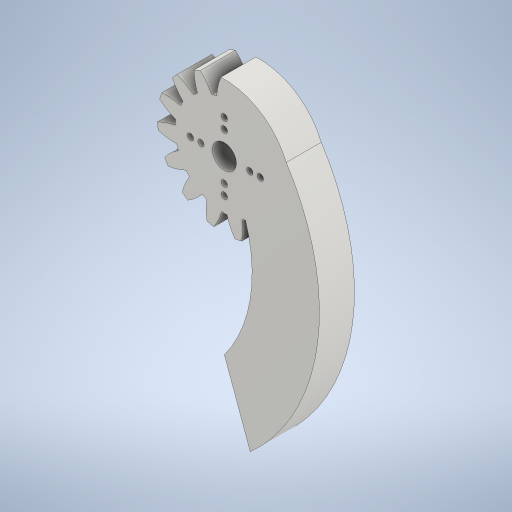
# Autodesk Inventor part: Spur Gear22
Saved by Autodesk Inventor 2024 (Build 280153000, 153)
## iProperties
CustomPartVersion: 0
Created: 2023-09-24
Part Number: Spur Gear22
Material: Steel
Document SubType Name: Modeling
Designer: jebes windows
Categories: <?xml version="1.0" encoding="UTF-16"?> <MemberInstance><Categories><FamilyTemplate><FamilyTemplateParameter ValueType="xs:double" Id="1" ObjectReferenceKey="da_z" ObjectType="kUserParameterObject"/><FamilyTemplateParameter ValueType="xs:double" Id="2" ObjectReferenceKey="da_b" ObjectType="kUserParameterObject"/><FamilyTemplateParameter ValueType="xs:double" Id="3" ObjectReferenceKey="da_beta" ObjectType="kUserParameterObject"/><FamilyTemplateParameter ValueType="xs:double" Id="4" ObjectReferenceKey="da_da" ObjectType="kUserParameterObject"/><FamilyTemplateParameter ValueType="xs:double" Id="5" ObjectReferenceKey="da_aw" ObjectType="kUserParameterObject"/><FamilyTemplateParameter ValueType="xs:string" Id="6" ObjectReferenceKey="EAIAABAAAACIAQAAAAAAAIAAAAAAAAAA" ObjectType="83910656" SubObjectId="SurfaceGeometry"/></FamilyTemplate><ParamToTemplateMap><ParamToTemplate CategoryParameter="//CategoryParameter[@InternalName='046C89C9-8512-4d59-83FE-43B91F4F132A']" TemplateParameter="1"/><ParamToTemplate CategoryParameter="//CategoryParameter[@InternalName='2552DF32-E462-4b46-AEBF-C6C7768E72AC']" TemplateParameter="2"/><ParamToTemplate CategoryParameter="//CategoryParameter[@InternalName='C9EE641D-15FC-4fae-A226-E94C4372FDD7']" TemplateParameter="3"/><ParamToTemplate><ParamToTemplate CategoryParameter="//CategoryParameter[@InternalName='00B6519A-459B-49c7-AD84-2E56D39A5744']" ConstantValue="0.102382"/></ParamToTemplate><ParamToTemplate><ParamToTemplate CategoryParameter="//CategoryParameter[@InternalName='04B31F0E-C7A6-4894-AA32-9629BEFACF47']" ConstantValue="1.000000"/></ParamToTemplate><ParamToTemplate><ParamToTemplate CategoryParameter="//CategoryParameter[@InternalName='43CBEC2E-7847-49e7-A936-2F7889FCB2D9']" ConstantValue="0.250000"/></ParamToTemplate><ParamToTemplate><ParamToTemplate CategoryParameter="//CategoryParameter[@InternalName='B1EFC894-105D-4ebd-86BF-FA20ED196853']" ConstantValue="0.302500"/></ParamToTemplate><ParamToTemplate><ParamToTemplate CategoryParameter="//CategoryParameter[@InternalName='51175063-3D10-4879-93E8-6246FE8B403D']" ConstantValue="2060000000.000000"/></ParamToTemplate><ParamToTemplate><ParamToTemplate CategoryParameter="//CategoryParameter[@InternalName='A3A52E27-4454-46a9-B0BD-C932399B70AF']" ConstantValue="0.300000"/></ParamToTemplate><ParamToTemplate><ParamToTemplate CategoryParameter="//CategoryParameter[@InternalName='91B76062-C214-41d9-B1B9-14D2AB99603D']" ConstantValue="0.150000"/></ParamToTemplate><ParamToTemplate><ParamToTemplate CategoryParameter="//CategoryParameter[@InternalName='374E806E-8B8A-4dda-A9AA-1039D6500AD2']" ConstantValue="6.666667"/></ParamToTemplate><ParamToTemplate><ParamToTemplate CategoryParameter="//CategoryParameter[@InternalName='2D373A89-B862-43d6-8D0B-0CBF12AB9F6C']" ConstantValue="0.349066"/></ParamToTemplate><ParamToTemplate CategoryParameter="//CategoryParameter[@InternalName='37777632-D6A2-4fac-9D53-DB8ACD95C989']" TemplateParameter="4"/><ParamToTemplate CategoryParameter="//CategoryParameter[@InternalName='FD1017F1-B727-4f7e-9707-0F86F1FF9423']" TemplateParameter="5"/><ParamToTemplate><ParamToTemplate CategoryParameter="//CategoryParameter[@InternalName='9E1B4470-B2D3-4ff1-B813-535BB4CDF51A']" ConstantValue="3520000.000000"/></ParamToTemplate><ParamToTemplate><ParamToTemplate CategoryParameter="//CategoryParameter[@InternalName='F8452263-BFF6-458c-9FB1-07C4B99E95CD']" ConstantValue="11400000.000000"/></ParamToTemplate><ParamToTemplate><ParamToTemplate CategoryParameter="//CategoryParameter[@InternalName='3E3BB259-FD49-497f-8171-6EBC954A3479']" ConstantValue="2.000000"/></ParamToTemplate><ParamToTemplate CategoryParameter="//CategoryParameter[@InternalName='27C3BAF2-7550-4e4b-AE2C-0DB134B7D9B7']" TemplateParameter="6"/></ParamToTemplateMap><Category DisplayName="Gear" InternalName="DC85795E-93AB-48d5-8EEE-5A27447B64BD" Mnemonic="Gear"><CategoryParameter DisplayName="z" InternalName="046C89C9-8512-4d59-83FE-43B91F4F132A" Mnemonic="z"/><CategoryParameter DisplayName="b" InternalName="2552DF32-E462-4b46-AEBF-C6C7768E72AC" Mnemonic="b"/><CategoryParameter DisplayName="||b|" InternalName="C9EE641D-15FC-4fae-A226-E94C4372FDD7" Mnemonic="beta"/><CategoryParameter DisplayName="x" InternalName="00B6519A-459B-49c7-AD84-2E56D39A5744" Mnemonic="x"/><CategoryParameter DisplayName="a*" InternalName="04B31F0E-C7A6-4894-AA32-9629BEFACF47" Mnemonic="a"/><CategoryParameter DisplayName="c*" InternalName="43CBEC2E-7847-49e7-A936-2F7889FCB2D9" Mnemonic="c"/><CategoryParameter DisplayName="r|.f|*" InternalName="B1EFC894-105D-4ebd-86BF-FA20ED196853" Mnemonic="rf"/><CategoryParameter DisplayName="E" InternalName="51175063-3D10-4879-93E8-6246FE8B403D" Mnemonic="E"/><CategoryParameter DisplayName="||m|" InternalName="A3A52E27-4454-46a9-B0BD-C932399B70AF" Mnemonic="mi"/><Category DisplayName="SpurGear" InternalName="26C5A22E-A91E-4dfd-A3B3-23CCAFAE1764" Mnemonic="SpurGear"><CategoryParameter DisplayName="m" InternalName="91B76062-C214-41d9-B1B9-14D2AB99603D" Mnemonic="m"/><CategoryParameter DisplayName="P" InternalName="374E806E-8B8A-4dda-A9AA-1039D6500AD2" Mnemonic="PP"/><CategoryParameter DisplayName="||a|" InternalName="2D373A89-B862-43d6-8D0B-0CBF12AB9F6C" Mnemonic="alpha"/><CategoryParameter DisplayName="d|.a|" InternalName="37777632-D6A2-4fac-9D53-DB8ACD95C989" Mnemonic="da"/><CategoryParameter DisplayName="a|.w|" InternalName="FD1017F1-B727-4f7e-9707-0F86F1FF9423" Mnemonic="aw"/><CategoryParameter DisplayName="||s||.Flim|" InternalName="9E1B4470-B2D3-4ff1-B813-535BB4CDF51A" Mnemonic="sFlim"/><CategoryParameter DisplayName="||s||.Hlim|" InternalName="F8452263-BFF6-458c-9FB1-07C4B99E95CD" Mnemonic="sHlim"/><CategoryParameter DisplayName="type" InternalName="3E3BB259-FD49-497f-8171-6EBC954A3479" Mnemonic="type"/><CategoryParameter DisplayName="PitchDiameter" InternalName="27C3BAF2-7550-4e4b-AE2C-0DB134B7D9B7" Mnemonic="IDS_PITCHDIAM"/></Category></Category></Categories></MemberInstance>
Density: 1 g/cm^3
Appearance: Steel
d16: 23,400 mm
d17: 0,000 mm
d41: 0,000 mm
d43: 23,400 mm
d46: 23,400 mm
d47: 0,000 mm
d48: 0,000 mm
Author: jebes windows
## iProperties of the stored document Spur Gear21_3DPrint.ipt
Created: 2023-09-24
Part Number: Spur Gear21_3DPrint
Material: Generic
Document SubType Name: Modeling
Designer: jebes windows
Density: 1 g/cm^3
Appearance: Default
Author: jebes windows
Autodesk Inventor part; units mm, degrees
ref_plane "YZ Plane" through (0, 0, 0) normal (1, 0, 0) x (0, 1, 0)
ref_plane "XZ Plane" through (0, 0, 0) normal (0, 1, 0) x (-1, 0, 0)
ref_plane "XY Plane" through (0, 0, 0) normal (0, 0, 1) x (1, 0, 0)
sketch "Sketch1" plane through (0, 0, 0) normal (0, 0, 1) x (1, 0, 0)
  circle A0 centre (0, 0) radius 12.745
  dimension "d0" = 25.49
  constraints: 1 centre point
  measures "d0" diameter of A0
extrude "Extrusion1" add sketch "Sketch1" along normal blind 6.6667
ref_plane "Work Plane2" through (0, 0, 3.3333) normal (0, 0, 1) x (1, 0, 0)
sketch "Sketch2" plane through (0, 0, 0) normal (0, 0, -1) x (-1, 0, 0)
  circle A0 centre (0, 0) radius 12.745 projected
  circle A1 centre (0, 0) radius 11.25
  dimension "d3" = 22.5
  constraints: 1 centre point, 1 coincident
  measures "d3" diameter of A1
surface extrude "Pitch Diameter" sketch "Sketch2" against normal through all shown no curves A1
ref_plane "Work Plane8" through (0, 0, 0) normal (0.9781476, 0.2079117, 0) x (0, 0, 1)
ref_plane "Work Plane9" through (0, 0, 0) normal (1, 0, 0) x (0, 1, 0)
spur gear teeth "Spur Gear" teeth 15 pitch diameter 22.5 tip diameter 25.49 root diameter 18.75 face width 10 start plane through (0, 0, 0) normal (0, 0, -1) x (-1, 0, 0)
sketch "Sketch3" plane through (0, 0, 0) normal (0, 0, -1) x (-1, 0, 0)
  line L0 (1.9, -6.45) -> (1.9, -2.8797) projected
  arc A0 (1.9, -2.8797) -> (2.2091, -2.65) centre (0, 0) ccw projected
  line L1 (2.2091, -2.65) -> (14.1591, -1.997) projected
  arc A1 (14.1591, -1.997) -> (14.1591, 1.997) centre (14.05, 0) ccw projected
  line L2 (14.1591, 1.997) -> (2.2091, 2.65) projected
  arc A2 (2.2091, 2.65) -> (1.9, 2.8797) centre (0, 0) ccw projected
  line L3 (1.9, 2.8797) -> (1.9, 6.45) projected
  arc A3 (1.9, 6.45) -> (-1.9, 6.45) centre (0, 6.45) ccw projected
  line L4 (-1.9, 6.45) -> (-1.9, 3.2953) projected
  line L5 (-1.9, 3.2953) -> (-16.6263, 1.9922) projected
  arc A4 (-16.6263, 1.9922) -> (-16.6263, -1.9922) centre (-16.45, 0) ccw projected
  line L6 (-16.6263, -1.9922) -> (-1.9, -3.2953) projected
  line L7 (-1.9, -3.2953) -> (-1.9, -6.45) projected
  arc A5 (-1.9, -6.45) -> (1.9, -6.45) centre (0, -6.45) ccw projected
  circle A6 centre (-14.85, 0) radius 0.6 projected
  circle A7 centre (-16.85, 0) radius 0.6 projected
  circle A8 centre (-12.85, 0) radius 0.6 projected
  circle A9 centre (-10.85, 0) radius 0.6 projected
  circle A10 centre (-8.85, 0) radius 0.6 projected
  circle A11 centre (-6.85, 0) radius 0.6 projected
  circle A12 centre (-4.85, 0) radius 0.6 projected
  circle A13 centre (4.45, 0) radius 0.6 projected
  circle A14 centre (6.45, 0) radius 0.6 projected
  circle A15 centre (8.45, 0) radius 0.6 projected
  circle A16 centre (10.45, 0) radius 0.6 projected
  circle A17 centre (14.45, 0) radius 0.6 projected
  circle A18 centre (12.45, 0) radius 0.6 projected
  circle A19 centre (0, 0) radius 2.3 projected
  circle A20 centre (0, -4.45) radius 0.6 projected
  circle A21 centre (0, -6.45) radius 0.6 projected
  circle A22 centre (0, 4.45) radius 0.6 projected
  circle A23 centre (0, 6.45) radius 0.6 projected
  point P0 (0, 0)
extrude "Extrusion2" cut sketch "Sketch3" against normal blind 10 contours A11 | A12 | A13 | A14 | A19 | A20 | A21 | A22 | A23
sketch "Sketch4" plane through (0, 0, 6.6667) normal (0, 0, 1) x (1, 0, 0)
  circle A0 centre (0, 0) radius 2.3 projected
  circle A1 centre (0, 6.45) radius 0.6 projected
  circle A2 centre (0, -4.45) radius 0.6 projected
  circle A3 centre (-4.45, 0) radius 0.6 projected
  circle A4 centre (6.85, 0) radius 0.6 projected
  circle A5 centre (0, 4.45) radius 0.6 projected
  circle A6 centre (0, -6.45) radius 0.6 projected
  circle A7 centre (-6.45, 0) radius 0.6 projected
  circle A8 centre (4.85, 0) radius 0.6 projected
  arc A9 (-4.5674, 11.8985) -> (-5.7861, 11.3559) centre (0, 0) ccw projected
  line L0 (0, 0) -> (0, -50)
  circle A10 centre (-21.7415, -16.631) radius 39.8269
  circle A11 centre (-21.7415, -16.631) radius 27.0188
  line L1 (0, -32.6723) -> (4.9275, -46.2105)
  arc A12 (-5.7861, 11.3559) -> (-5.106, 7.8625) centre (4.8082, 11.6056) ccw projected
  arc A13 (-5.106, 7.8625) -> (-5.8999, 7.2857) centre (0, 0) ccw projected
  arc A14 (-5.8999, 7.2857) -> (-9.0121, 9.0121) centre (-12.5234, -0.9865) ccw projected
  arc A15 (-9.0121, 9.0121) -> (-9.9047, 8.0207) centre (0, 0) ccw projected
  arc A16 (-9.9047, 8.0207) -> (-7.8625, 5.106) centre (-0.3279, 12.5579) ccw projected
  arc A17 (-7.8625, 5.106) -> (-8.3532, 4.2562) centre (0, 0) ccw projected
  arc A18 (-8.3532, 4.2562) -> (-11.8985, 4.5674) centre (-11.0394, -5.995) ccw projected
  arc A19 (-11.8985, 4.5674) -> (-12.3107, 3.2986) centre (0, 0) ccw projected
  arc A20 (-12.3107, 3.2986) -> (-9.2596, 1.4666) centre (-5.4073, 11.3388) ccw projected
  arc A21 (-9.2596, 1.4666) -> (-9.3622, 0.4906) centre (0, 0) ccw projected
  arc A22 (-9.3622, 0.4906) -> (-12.7275, -0.667) centre (-7.6467, -9.9668) ccw projected
  arc A23 (-12.7275, -0.667) -> (-12.5881, -1.9938) centre (0, 0) ccw projected
  arc A24 (-12.5881, -1.9938) -> (-9.0556, -2.4264) centre (-9.5518, 8.1592) ccw projected
  arc A25 (-9.0556, -2.4264) -> (-8.7523, -3.3597) centre (0, 0) ccw projected
  arc A26 (-8.7523, -3.3597) -> (-11.3559, -5.7861) centre (-2.9317, -12.2153) ccw projected
  arc A27 (-11.3559, -5.7861) -> (-10.6889, -6.9414) centre (0, 0) ccw projected
  arc A28 (-10.6889, -6.9414) -> (-7.2857, -5.8999) centre (-12.0446, 3.5687) ccw projected
  arc A29 (-7.2857, -5.8999) -> (-6.6291, -6.6291) centre (0, 0) ccw projected
  arc A30 (-6.6291, -6.6291) -> (-8.0207, -9.9047) centre (2.2902, -12.3517) ccw projected
  arc A31 (-8.0207, -9.9047) -> (-6.9414, -10.6889) centre (0, 0) ccw projected
  arc A32 (-6.9414, -10.6889) -> (-4.2562, -8.3532) centre (-12.4548, -1.6388) ccw projected
  arc A33 (-4.2562, -8.3532) -> (-3.3597, -8.7523) centre (0, 0) ccw projected
  arc A34 (-3.3597, -8.7523) -> (-3.2986, -12.3107) centre (7.1161, -10.3523) ccw projected
  arc A35 (-3.2986, -12.3107) -> (-1.9938, -12.5881) centre (0, 0) ccw projected
  arc A36 (-1.9938, -12.5881) -> (-0.4906, -9.3622) centre (-10.7115, -6.5629) ccw projected
  arc A37 (-0.4906, -9.3622) -> (0.4906, -9.3622) centre (0, 0) ccw projected
  arc A38 (0.4906, -9.3622) -> (1.9938, -12.5881) centre (10.7115, -6.5629) ccw projected
  arc A39 (1.9938, -12.5881) -> (3.2986, -12.3107) centre (0, 0) ccw projected
  arc A40 (3.2986, -12.3107) -> (3.3597, -8.7523) centre (-7.1161, -10.3523) ccw projected
  arc A41 (3.3597, -8.7523) -> (4.2562, -8.3532) centre (0, 0) ccw projected
  arc A42 (4.2562, -8.3532) -> (6.9414, -10.6889) centre (12.4548, -1.6388) ccw projected
  arc A43 (6.9414, -10.6889) -> (8.0207, -9.9047) centre (0, 0) ccw projected
  arc A44 (8.0207, -9.9047) -> (6.6291, -6.6291) centre (-2.2902, -12.3517) ccw projected
  arc A45 (6.6291, -6.6291) -> (7.2857, -5.8999) centre (0, 0) ccw projected
  arc A46 (7.2857, -5.8999) -> (10.6889, -6.9414) centre (12.0446, 3.5687) ccw projected
  arc A47 (10.6889, -6.9414) -> (11.3559, -5.7861) centre (0, 0) ccw projected
  arc A48 (11.3559, -5.7861) -> (8.7523, -3.3597) centre (2.9317, -12.2153) ccw projected
  arc A49 (8.7523, -3.3597) -> (9.0556, -2.4264) centre (0, 0) ccw projected
  arc A50 (9.0556, -2.4264) -> (12.5881, -1.9938) centre (9.5518, 8.1592) ccw projected
  arc A51 (12.5881, -1.9938) -> (12.7275, -0.667) centre (0, 0) ccw projected
  arc A52 (12.7275, -0.667) -> (9.3622, 0.4906) centre (7.6467, -9.9668) ccw projected
  arc A53 (9.3622, 0.4906) -> (9.2596, 1.4666) centre (0, 0) ccw projected
  arc A54 (9.2596, 1.4666) -> (12.3107, 3.2986) centre (5.4073, 11.3388) ccw projected
  arc A55 (12.3107, 3.2986) -> (11.8985, 4.5674) centre (0, 0) ccw projected
  arc A56 (11.8985, 4.5674) -> (8.3532, 4.2562) centre (11.0394, -5.995) ccw projected
  arc A57 (8.3532, 4.2562) -> (7.8625, 5.106) centre (0, 0) ccw projected
  arc A58 (7.8625, 5.106) -> (9.9047, 8.0207) centre (0.3279, 12.5579) ccw projected
  arc A59 (9.9047, 8.0207) -> (9.0121, 9.0121) centre (0, 0) ccw projected
  arc A60 (9.0121, 9.0121) -> (5.8999, 7.2857) centre (12.5234, -0.9865) ccw projected
  arc A61 (5.8999, 7.2857) -> (5.106, 7.8625) centre (0, 0) ccw projected
  arc A62 (5.106, 7.8625) -> (5.7861, 11.3559) centre (-4.8082, 11.6056) ccw projected
  arc A63 (5.7861, 11.3559) -> (4.5674, 11.8985) centre (0, 0) ccw projected
  arc A64 (4.5674, 11.8985) -> (2.4264, 9.0556) centre (11.842, 4.1925) ccw projected
  arc A65 (2.4264, 9.0556) -> (1.4666, 9.2596) centre (0, 0) ccw projected
  arc A66 (1.4666, 9.2596) -> (0.667, 12.7275) centre (-9.1129, 8.6466) ccw projected
  arc A67 (0.667, 12.7275) -> (-0.667, 12.7275) centre (0, 0) ccw projected
  arc A68 (-0.667, 12.7275) -> (-1.4666, 9.2596) centre (9.1129, 8.6466) ccw projected
  arc A69 (-1.4666, 9.2596) -> (-2.4264, 9.0556) centre (0, 0) ccw projected
  arc A70 (-2.4264, 9.0556) -> (-4.5674, 11.8985) centre (-11.842, 4.1925) ccw projected
  circle A71 centre (0, 0) radius 12.745
  point P0 (-1.8858, -13.5191)
  point P1 (14.304, 0.3073)
  point P2 (0, -0.5897)
  point P3 (4.5674, 11.8985)
  point P4 (0.667, 12.7275)
  point P5 (9.0121, 9.0121)
  point P6 (5.7861, 11.3559)
  point P7 (11.7685, 4.8925)
  point P8 (9.9047, 8.0207)
  point P9 (4.0158, -8.4714)
  dimension "d53" = 54.0377
  dimension "d51" = 50
  dimension "d52" = 79.6539
  dimension "d61" = 20
  dimension "d62" = 21.7415
  dimension "d63" = 27.373
  dimension "d65" = 4.85
  dimension "d66" = 16.631
  constraints: 4 end point, 3 point on circle, 2 centre point, 1 coincident, 1 concentric, 1 point on line, 1 vertical, 3 other
  measures "d51" distance of L0.start L0.end
  measures "d52" diameter of A10
  measures "d61" angle of L0 L1
  measures "d62" horizontal distance of point (0, 0) A10.centre
  measures "d63" distance of A0.centre A10.centre
  measures "d65" distance from line of L0 A8.centre
  measures "d66" vertical distance of A10.centre A0.centre
extrude "Extrusion3" add sketch "Sketch4" against normal blind 6.6667 contours A41 A42 A71 A11 | A71 A43 A47 A51 A55 A10 L1 A11 | A44 A45 A46 A71 | A71 A60 A10 | A10 A60 A61 A62 A71 | A71 A56 A57 A58 A10 | A10 A58 A71 | A48 A49 A50 A71 | A64 A65 A66 A71 | A71 A52 A53 A54
equation "\"d0\" = da_da"
equation "\"d1\" = 0.666667 * da_b"
equation "\"d16\" = da_aw"
equation "\"d54\" = 0.666667 * da_b"
equation "\"d3\" = da_d"
equation "\"d43\" = da_aw"
equation "\"d46\" = da_aw"
equation "\"da_da\" = 25.49"
equation "\"da_b\" = 10"
equation "\"da_aw\" = 23.4"
equation "\"da_d\" = 22.5"
body "Solid1"
body "Srf1"
